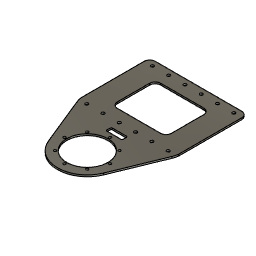
JumperTrunk_MidPlates v2 (Autodesk Fusion 360 design; units mm, degrees)
Autodesk Fusion 360 part; units mm, degrees
sketch "Sketch1" plane through (0, 0, 0) normal (0, 0, 1) x (1, 0, 0)
  line L0 (180, 133.6216) -> (180, 250)
  line L1 (170, 260) -> (10, 260)
  line L2 (0, 250) -> (0, 133.4829)
  circle A0 centre (90.016, 55) radius 38
  circle A1 centre (90.016, 55) radius 42 construction
  line L3 (2.627, 123.5637) -> (39.0941, 34.2163)
  line L4 (177.3504, 123.503) -> (140.9438, 34.2308)
  arc A2 (0, 133.4829) -> (2.627, 123.5637) centre (39.6611, 138.6792) ccw
  arc A3 (177.3504, 123.503) -> (180, 133.6216) centre (140.312, 138.6078) ccw
  arc A4 (10, 260) -> (0, 250) centre (10, 250) ccw
  arc A5 (180, 250) -> (170, 260) centre (170, 250) ccw
  arc A6 (39.0941, 34.2163) -> (140.9438, 34.2308) centre (90.016, 55) ccw
  circle A7 centre (90, 97) radius 2.25
  circle A8 centre (60.3062, 84.6872) radius 2.25
  circle A9 centre (48.016, 54.984) radius 2.25
  circle A10 centre (60.3288, 25.2902) radius 2.25
  circle A11 centre (90.032, 13) radius 2.25
  circle A12 centre (119.7258, 25.3128) radius 2.25
  circle A13 centre (132.016, 55.016) radius 2.25
  circle A14 centre (119.7032, 84.7098) radius 2.25
  line L5 (77.016, 104) -> (103.016, 104)
  line L6 (105.016, 106) -> (105.016, 112)
  line L7 (103.016, 114) -> (77.016, 114)
  line L8 (75.016, 112) -> (75.016, 106)
  arc A15 (77.016, 114) -> (75.016, 112) centre (77.016, 112) ccw
  arc A16 (75.016, 106) -> (77.016, 104) centre (77.016, 106) ccw
  arc A17 (103.016, 104) -> (105.016, 106) centre (103.016, 106) ccw
  arc A18 (105.016, 112) -> (103.016, 114) centre (103.016, 112) ccw
  circle A19 centre (15, 129) radius 2.75
  circle A20 centre (15, 250) radius 2.75
  circle A21 centre (45, 250) radius 2.75
  circle A22 centre (45, 129) radius 2.75
  circle A23 centre (75, 250) radius 2.75
  circle A24 centre (105, 250) radius 2.75
  circle A25 centre (135, 250) radius 2.75
  circle A26 centre (135, 129) radius 2.75
  circle A27 centre (165, 250) radius 2.75
  circle A28 centre (165, 129) radius 2.75
  line L9 (130, 150) -> (50, 150)
  line L10 (40, 160) -> (40, 220)
  line L11 (50, 230) -> (130, 230)
  line L12 (140, 220) -> (140, 160)
  arc A29 (50, 230) -> (40, 220) centre (50, 220) ccw
  arc A30 (140, 220) -> (130, 230) centre (130, 220) ccw
  arc A31 (130, 150) -> (140, 160) centre (130, 160) ccw
  arc A32 (40, 160) -> (50, 150) centre (50, 160) ccw
  circle A33 centre (75, 129) radius 2.75
  circle A34 centre (105, 129) radius 2.75
  point P0 (180, 260)
  point P1 (0, 260)
  point P2 (0, 130)
  point P3 (75.016, 104)
  point P4 (105.016, 114)
  point P5 (75.016, 114)
  dimension "d1" = 260
  dimension "d3" = 76
  dimension "d4" = 84
  dimension "d5" = 110
  dimension "d8" = 130
  dimension "d9" = 180
  dimension "d10" = 40
  dimension "d11" = 10
  dimension "d12" = 4.5
  dimension "d13" = 90
  dimension "d15" = 360
  dimension "d32" = 30
  dimension "d33" = 10
  dimension "d34" = 15
  dimension "d35" = 49
  dimension "d36" = 2
  dimension "d37" = 5.5
  dimension "d38" = 15
  dimension "d39" = 5.5
  dimension "d40" = 15
  dimension "d41" = 10
  dimension "d44" = 30
  dimension "d45" = 0
  dimension "d48" = 80
  dimension "d49" = 30
  dimension "d50" = 10
  dimension "d57" = 15
  dimension "d60" = 60
  dimension "d61" = 0
  dimension "d65" = 40
  constraint vertical L0
  constraint horizontal L1
  constraint vertical L2
  constraint concentric A0 A1
  constraint concentric A1 A6
  constraint tangent L4 A6
  constraint tangent L3 A6
  constraint coincident P2 L3
  constraint coincident L2 P2
  constraint tangent L3 A2
  constraint tangent L4 A3
  constraint equal A2 A3
  constraint coincident P1 L1
  constraint coincident P1 L2
  constraint tangent L1 A4
  constraint tangent L2 A4
  constraint coincident P0 L0
  constraint coincident P0 L1
  constraint tangent L0 A5
  constraint tangent L1 A5
  constraint equal A4 A5
  constraint coincident A1 A7.centre
  constraint horizontal L5
  constraint vertical L6
  constraint horizontal L7
  constraint vertical L8
  constraint coincident P5 L7
  constraint coincident P5 L8
  constraint tangent L7 A15
  constraint tangent L8 A15
  constraint coincident P3 L5
  constraint coincident P3 L8
  constraint tangent L5 A16
  constraint tangent L8 A16
  constraint equal A15 A16
  constraint tangent L5 A17
  constraint tangent L6 A17
  constraint equal A15 A17
  constraint coincident P4 L6
  constraint coincident P4 L7
  constraint tangent L6 A18
  constraint tangent L7 A18
  constraint equal A15 A18
  constraint horizontal L9
  constraint vertical L10
  constraint horizontal L11
  constraint vertical L12
  constraint tangent L10 A29
  constraint tangent L11 A29
  constraint tangent L11 A30
  constraint tangent L12 A30
  constraint equal A29 A30
  constraint tangent L9 A31
  constraint tangent L12 A31
  constraint equal A29 A31
  constraint tangent L9 A32
  constraint tangent L10 A32
  constraint equal A29 A32
  measures "d1" distance of origin P1
  measures "d3" diameter of A0
  measures "d4" diameter of A1
  measures "d5" diameter of A6
  measures "d8" distance of origin P2
  measures "d9" distance of P0 P1
  measures "d10" radius of A2
  measures "d11" radius of A4
  measures "d12" diameter of A7
  measures "d13" distance of L2 A7.centre
  measures "d32" distance of P4 P5
  measures "d33" distance of P3 P5
  measures "d34" horizontal distance of A0.centre P3
  measures "d35" distance of A0.centre L5
  measures "d36" radius of A15
  measures "d37" diameter of A19
  measures "d38" distance of L2 A19.centre
  measures "d39" diameter of A20
  measures "d40" distance of L2 A20.centre
  measures "d41" distance of L1 A20.centre
  measures "d48" distance of L9 L11
  measures "d49" distance of L1 L11
  measures "d50" radius of A29
  measures "d57" distance of L7 A22.centre
  measures "d65" distance of L2 L10
extrude "Extrude1" add sketch "Sketch1" along normal blind 3 contours L0 L1 L2 L3 L4 A2 A3 A4 A5 A6 | A33 | A34
extrude "Extrude3" cut sketch "Sketch1" along normal through all contours A33 | A34
extrude "Extrude2" [suppressed]
